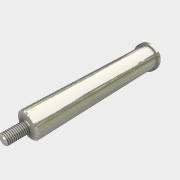
# Autodesk Inventor part: PWTR-0111
Saved by Autodesk Inventor 2021.1 (Build 251245000, 245)
## iProperties
Created: 2020-09-01
Part Number: PWTR-0111
Material: Stainless Steel
Document SubType Name: Modeling
Designer: alid
Density: 8 g/cm^3
Appearance: Titanium - Polished
Description: Arm Pivot Pin
Author: alid
Revision Number: A
Autodesk Inventor part; units mm, degrees
ref_plane "YZ Plane" through (0, 0, 0) normal (1, 0, 0) x (0, 1, 0)
ref_plane "XZ Plane" through (0, 0, 0) normal (0, 1, 0) x (-1, 0, 0)
ref_plane "XY Plane" through (0, 0, 0) normal (0, 0, 1) x (1, 0, 0)
sketch "Sketch1" plane through (0, 0, 0) normal (0, 0, 1) x (1, 0, 0)
  line L0 (-82.5, 0) -> (82.5, 0)
  line L1 (-82.5, 0) -> (-82.5, 12.5)
  line L2 (-82.5, 12.5) -> (77.5, 12.5)
  line L3 (77.5, 12.5) -> (77.5, 15)
  line L4 (77.5, 15) -> (82.5, 15)
  line L5 (82.5, 15) -> (82.5, 0)
  circle A0 centre (-72.5, 0) radius 1.75
  line L6 (77.5, 12.75) -> (57.5, 12.5)
  line L7 (-82.5, 5) -> (-62.5, 5)
  line L8 (-62.5, 5) -> (-62.5, 12.5)
  point P0 (0, 0)
  point P1 (0, 0)
  dimension "d0" = 165
  dimension "d1" = 25
  dimension "d2" = 5
  dimension "d3" = 30
  dimension "d8" = 3.5
  dimension "d9" = 10
  dimension "d12" = 0.25
  dimension "d13" = 20
  dimension "d14" = 10
  dimension "d15" = 20
  constraints: 18 end point, 5 perpendicular, 5 point on line, 1 centre point, 1 coincident, 1 horizontal, 1 midpoint, 1 vertical
  measures "d0" distance of L0.start L0.end
  measures "d1" diameter of L2 L0
  measures "d2" distance of L3.end L4.end
  measures "d3" diameter of L4 L0
  measures "d8" diameter of A0
  measures "d9" distance from line of L1 A0.centre
  measures "d12" distance from line of L2 L6.start
  measures "d13" horizontal distance of L6.start L6.end
  measures "d14" diameter of L7 L0
  measures "d15" distance of L7.start L7.end
revolve "Revolution1" add sketch "Sketch1" angle 360 about axis through (-82.5, 0, 0) along (1, 0, 0) picked at (-71.9665, 0.4107) contours A0 L0 L1 L7 L8 L2 L3 L4 L5 | L0 A0 | L3 L2 L6
fillet "Fillet1" radius 1 1 edges at (-62.5, -5, 0)
thread "Thread1" size "M10x1.5" class "6g" standard "ISO Metric profile" full length
chamfer "Chamfer1" distance 1 angle 45 3 edges at (82.5, -15, 0) (-62.5, -12.5, 0) (-82.5, -5, 0)
body "Solid1"
